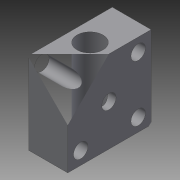
# Autodesk Inventor part: Tube Bracket
Saved by Autodesk Inventor 2014 SP1 (Build 180222100, 222)
## iProperties
Created: 2014-01-22
Part Number: Tube Bracket
Material: Generic
Document SubType Name: Modeling
Designer: tom
Density: 1 g/cm^3
Appearance: Default
Author: tom
Autodesk Inventor part; units mm, degrees
ref_plane "YZ Plane" through (0, 0, 0) normal (1, 0, 0) x (0, 1, 0)
ref_plane "XZ Plane" through (0, 0, 0) normal (0, 1, 0) x (-1, 0, 0)
ref_plane "XY Plane" through (0, 0, 0) normal (0, 0, 1) x (1, 0, 0)
sketch "Sketch1" plane through (0, 0, 0) normal (1, 0, 0) x (0, 1, 0)
  circle A0 centre (-6.9088, 6.9088) radius 1.778
  circle A1 centre (6.9088, 6.9088) radius 1.778
  circle A2 centre (-6.9088, -7.1628) radius 1.778
  circle A3 centre (6.9088, -7.1628) radius 1.778
  line L0 (-10.0838, 10.0838) -> (10.0838, 10.0838)
  line L1 (10.0838, 10.0838) -> (10.0838, -10.3378)
  line L2 (10.0838, -10.3378) -> (-10.0838, -10.3378)
  line L3 (-10.0838, -10.3378) -> (-10.0838, 10.0838)
  point P0 (0, 0)
  dimension "d0" = 6.9088
  dimension "d1" = 6.9088
  dimension "d2" = 13.8176
  dimension "d3" = 14.0716
  dimension "d4" = 3.556
  dimension "d5" = 3.556
  dimension "d6" = 3.556
  dimension "d7" = 3.556
  dimension "d8" = 3.175
  dimension "d9" = 3.175
  dimension "d10" = 3.175
  dimension "d11" = 3.175
  constraints: 8 end point, 4 centre point, 2 parallel, 1 horizontal, 1 perpendicular
  measures "d0" horizontal distance of point (0, 0) A0.centre
  measures "d1" horizontal distance of point (0, 0) A0.centre
  measures "d2" distance of A1.centre A0.centre
  measures "d3" distance of A2.centre A0.centre
  measures "d4" diameter of A3
  measures "d5" diameter of A2
  measures "d6" diameter of A0
  measures "d7" diameter of A1
  measures "d8" distance from line of L3 A0.centre
  measures "d9" distance from line of L1 A1.centre
  measures "d10" distance from line of L0 A0.centre
  measures "d11" distance from line of L2 A2.centre
extrude "Extrusion1" add sketch "Sketch1" along normal blind 9.525
sketch "Sketch2" plane through (0, 10.0838, 10.0838) normal (0, 1, 0) x (1, 0, 0)
  circle A0 centre (4.7625, 10.2108) radius 3.175
  line L0 (0, 0) -> (0, 20.4216) projected
  line L1 (0, 20.4216) -> (9.525, 20.4216) projected
  point P0 (0, 10.0838)
  dimension "d14" = 6.35
  dimension "d17" = 4.7625
  dimension "d18" = 10.2108
  constraints: 1 centre point
  measures "d14" diameter of A0
  measures "d17" distance from line of A0.centre L0
  measures "d18" distance from line of L1 A0.centre
extrude "Extrusion2" cut sketch "Sketch2" against normal blind 38.1
sketch "Sketch3" plane through (9.525, 0, 0) normal (1, 0, 0) x (0, 0, -1)
  circle A0 centre (0, 0) radius 1.7526
  dimension "d19" = 3.5052
  constraints: 1 centre point, 1 coincident
  measures "d19" diameter of A0
extrude "Extrusion3" cut sketch "Sketch3" against normal blind 4.7625
body "Solid1"
